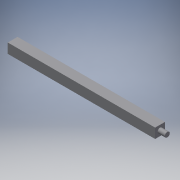
# Autodesk Inventor part: hopper_bar
Saved by Autodesk Inventor 2017 (Build 210142000, 142)
## iProperties
Created: 2020-01-18
Part Number: hopper_bar
Material: Generic
Document SubType Name: Modeling
Designer: S338578040
Density: 1 g/cm^3
Appearance: Default
Author: S338578040
Autodesk Inventor part; units mm, degrees
ref_plane "YZ Plane" through (0, 0, 0) normal (1, 0, 0) x (0, 1, 0)
ref_plane "XZ Plane" through (0, 0, 0) normal (0, 1, 0) x (-1, 0, 0)
ref_plane "XY Plane" through (0, 0, 0) normal (0, 0, 1) x (1, 0, 0)
sketch "Sketch1" plane through (0, 0, 0) normal (1, 0, 0) x (0, 1, 0)
  line L0 (0, 0) -> (-25.4, 0)
  line L1 (-25.4, 0) -> (-25.4, -25.4)
  line L2 (-25.4, -25.4) -> (0, -25.4)
  line L3 (0, -25.4) -> (0, 0)
  dimension "d0" = 25.4
  dimension "d1" = 25.4
  constraints: 8 end point, 2 parallel, 1 horizontal, 1 perpendicular
  measures "d0" distance of L2.end L0.start
  measures "d1" distance of L0.start L0.end
extrude "Extrusion1" add sketch "Sketch1" along normal blind 406.4
sketch "Sketch2" plane through (406.4, 0, 0) normal (1, 0, 0) x (0, 0, -1)
  circle A0 centre (12.7, -12.7) radius 6.35
  line L0 (12.7, -12.7) -> (12.7, 0) construction
  line L1 (25.4, 0) -> (0, 0) projected
  dimension "d4" = 12.7
  dimension "d11" = 12.7
  constraints: 2 end point, 1 centre point, 1 midpoint
  measures "d4" diameter of A0
  measures "d11" distance of L0.start L0.end
extrude "Extrusion2" add sketch "Sketch2" along normal blind 18.796
sketch "Sketch3" plane through (0, 0, 0) normal (-1, 0, 0) x (0, 0, 1)
  circle A0 centre (-12.7, -12.7) radius 6.35
  line L0 (-12.7, -12.7) -> (-12.7, 0) construction
  line L1 (-25.4, 0) -> (0, 0) construction
  line L2 (0, 0) -> (0, -25.4) construction
  dimension "d9" = 12.7
  dimension "d10" = 12.7
  constraints: 2 end point, 1 centre point, 1 midpoint, 1 parallel
  measures "d9" diameter of A0
  measures "d10" distance of L0.start L0.end
extrude "Extrusion3" add sketch "Sketch3" against normal blind 19.05
sketch "Sketch4" plane through (0, -25.4, 0) normal (0, 0, 1) x (1, 0, 0)
  line L0 (0, 25.4) -> (403.86, 25.4)
  line L1 (403.86, 25.4) -> (403.86, 30.48)
  line L2 (403.86, 30.48) -> (0, 30.48)
  line L3 (0, 30.48) -> (0, 25.4)
  dimension "d12" = 5.08
  dimension "d15" = 403.86
  constraints: 8 end point, 2 parallel, 1 horizontal, 1 perpendicular
  measures "d12" distance of L1.end L0.end
  measures "d15" distance of L1.end L2.end
extrude "Extrusion4" add sketch "Sketch4" against normal blind 177.8
body "Solid1"
